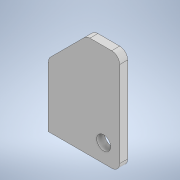
# Autodesk Inventor part: ScrewStopper
Saved by Autodesk Inventor 2022 (Build 260153000, 153)
## iProperties
Created: 2021-11-15
Part Number: ScrewStopper
Material: Generic
Document SubType Name: Modeling
Designer: lgnds
Density: 1 g/cm^3
Appearance: Default
Author: lgnds
Autodesk Inventor part; units mm, degrees
ref_plane "YZ Plane" through (0, 0, 0) normal (1, 0, 0) x (0, 1, 0)
ref_plane "XZ Plane" through (0, 0, 0) normal (0, 1, 0) x (-1, 0, 0)
ref_plane "XY Plane" through (0, 0, 0) normal (0, 0, 1) x (1, 0, 0)
sketch "Sketch1" plane through (0, 0, 0) normal (0, 0, 1) x (1, 0, 0)
  line L0 (0, 0) -> (0, 25.452)
  line L1 (0, 25.452) -> (-8.276, 25.452)
  line L2 (-8.276, 25.452) -> (-18, 15.728)
  line L3 (-18, 15.728) -> (-18, 0)
  line L4 (-18, 0) -> (0, 0)
  dimension "d0" = 8.276
  dimension "d1" = 18
  dimension "d2" = 135
  dimension "d3" = 25.452
  constraints: 10 end point, 2 perpendicular, 1 parallel, 1 vertical
  measures "d0" distance of L0.end L1.end
  measures "d1" distance between parallel lines of L0 L3
  measures "d2" angle of L1 L2
  measures "d3" distance between parallel lines of L4 L1
extrude "Extrusion1" add sketch "Sketch1" along normal blind 2
sketch "Sketch2" plane through (0, 0, 2) normal (0, 0, 1) x (1, 0, 0)
  line L0 (0, 25.452) -> (-8.276, 25.452) projected
  line L1 (-8.276, 25.452) -> (-18, 15.728) projected
  line L2 (-18, 15.728) -> (-18, 0) projected
  line L3 (-18, 0) -> (0, 0) projected
  line L4 (0, 0) -> (0, 25.452) projected
  line L5 (-18, 0) -> (0, 0) projected
  line L6 (-14, 0) -> (-14, 3)
  arc A0 (-14, 3) -> (-18, 3) centre (-16, 3) ccw
  dimension "d6" = 4
  dimension "d7" = 3
  dimension "d8" = 2
  constraints: 2 end point, 2 point on circle, 2 point on line, 1 centre point, 1 tangent, 1 vertical
  measures "d6" distance between parallel lines of L2 L6
  measures "d7" distance of L6.start L6.end
  measures "d8" radius of A0
extrude "Extrusion2" add sketch "Sketch2" against normal blind 3 contours L3 L2 A0 L6
sketch "Sketch7" plane through (0, 0, -1) normal (0, 0, -1) x (-1, 0, 0)
  line L0 (18, 0) -> (18, 3) projected
  arc A0 (18, 3) -> (14, 3) centre (16, 3) ccw projected
  line L1 (14, 3) -> (14, 0) projected
  line L2 (14, 0) -> (18, 0) projected
  arc A1 (17.85, 3) -> (14.15, 3) centre (16, 3) ccw
  line L3 (17.85, 3) -> (17.85, 0.15)
  line L4 (17.85, 0.15) -> (14.15, 0.15)
  line L5 (14.15, 0.15) -> (14.15, 3)
  line L6 (14.15, 0.15) -> (14.15, 0)
  line L7 (17.85, 0.15) -> (17.85, 0)
  point P0 (0, 0)
  dimension "d24" = 0.15
  constraints: 10 end point, 2 point on circle, 2 point on line, 2 vertical, 1 centre point, 3 other
  measures "d24" distance between parallel lines of L1 L5
extrude "Extrusion6" cut sketch "Sketch7" against normal up to surface (1 mm away) contours L2 L7 L3 A1 L5 L6 L1 A0 L0
sketch "Sketch4" plane through (0, 0, 2) normal (0, 0, 1) x (1, 0, 0)
  circle A0 centre (-4, 4.5) radius 1.75
  line L0 (-18, 15.728) -> (-18, 0) projected
  line L1 (-18, 0) -> (0, 0) projected
  point P0 (-14.15, 0)
  point P1 (-18, 3)
  point P2 (-14, 0)
  dimension "d14" = 3.5
  dimension "d15" = 14
  dimension "d16" = 4.5
  constraints: 1 centre point
  measures "d14" diameter of A0
  measures "d15" distance from line of L0 A0.centre
  measures "d16" distance from line of L1 A0.centre
extrude "Extrusion4" cut sketch "Sketch4" against normal up to surface (2 mm away)
sketch "Sketch5" plane through (-18, 0, 0) normal (-1, 0, 0) x (0, 0, 1)
  line L0 (2, 15.728) -> (2, 0) projected
  line L1 (0, 15.728) -> (2, 15.728) projected
  line L2 (2, 0) -> (2, 25.452) projected
  line L3 (0, 15.728) -> (2, 15.728)
  line L4 (2, 15.728) -> (2, 19.0295)
  line L5 (2, 19.0295) -> (0, 19.0295)
  line L6 (0, 19.0295) -> (0, 15.728)
  line L7 (0, 15.728) -> (0, 0) projected
  line L8 (0, 0) -> (2, 0) projected
  point P0 (0, 0)
  constraints: 8 end point, 2 parallel, 1 horizontal, 1 perpendicular, 1 point on line
extrude "Extrusion5" cut sketch "Sketch5" against normal up to surface (0.15 mm away)
fillet "Fillet1" radius 2 4 edges at (-17.85, 15.878, 1) (-8.276, 25.452, 1) (0, 25.452, 1) (0, 0, 1)
sketch "Sketch6" plane through (0, 0, 2) normal (0, 0, 1) x (1, 0, 0)
  circle A0 centre (1.75, 1.9974) radius 1.5
  line L0 (0, 2) -> (0, 23.452) projected
  point P0 (0, 0)
  dimension "d22" = 3
  dimension "d23" = 1.75
  constraints: 1 centre point
  measures "d22" diameter of A0
  measures "d23" distance from line of L0 A0.centre
body "Solid1"
